Autodesk Fusion 360 part; units mm, degrees
(part 2 of 2)
sketch "스케치7" plane through (0, 0, -15.8) normal (0, 0, 1) x (-1, 0, 0) in component "right-body"
  arc A0 (-30.595085, -3.272852) -> (-28.095085, -5.772852) centre (-28.095085, -3.272852) ccw
  line L0 (-30.595085, -3.272852) -> (-218.195, -3.272852)
  arc A1 (-220.695, -5.772852) -> (-218.195, -3.272852) centre (-220.695, -3.272852) ccw
  line L1 (-220.695, -5.772852) -> (-220.695, -98.121)
  arc A2 (-218.195, -100.621) -> (-220.695, -98.121) centre (-220.695, -100.621) ccw
  line L2 (-218.195, -100.621) -> (-30.595085, -100.621)
  arc A3 (-28.095085, -98.121) -> (-30.595085, -100.621) centre (-28.095085, -100.621) ccw
  line L3 (-28.095085, -98.121) -> (-28.095085, -5.772852)
  line L4 (-30.595085, -100.621) -> (-30.595085, -3.272852)
  line L5 (-33.595085, -87.321) -> (-45.595085, -87.321)
  line L6 (-45.595085, -87.321) -> (-45.595085, -84.321)
  line L7 (-45.595085, -84.321) -> (-33.595085, -84.321)
  line L8 (-33.595085, -84.321) -> (-33.595085, -87.321)
  line L9 (-218.195, -100.621) -> (-30.595085, -100.621)
  line L10 (-58.595085, -65.221) -> (-76.595085, -65.221)
  line L11 (-76.595085, -65.221) -> (-76.595085, -62.221)
  line L12 (-76.595085, -62.221) -> (-58.595085, -62.221)
  line L13 (-58.595085, -62.221) -> (-58.595085, -65.221)
  line L14 (-59.9071, -58.8987) -> (-59.9071, -44.9972)
  line L15 (-65.0569, -44.9972) -> (-65.0569, -58.8987)
  line L16 (-78.957, -58.8987) -> (-78.957, -44.9972)
  line L17 (-84.1069, -44.9972) -> (-84.1069, -58.8987)
  line L18 (-98.007, -58.8987) -> (-98.007, -44.9972)
  line L19 (-103.1569, -44.9972) -> (-103.1569, -58.8987)
  line L20 (-117.057, -58.8987) -> (-117.057, -44.9972)
  line L21 (-122.2069, -44.9972) -> (-122.2069, -58.8987)
  line L22 (-136.107, -58.8987) -> (-136.107, -44.9972)
  line L23 (-141.257, -44.9972) -> (-141.257, -58.8987)
  line L24 (-155.157, -58.8987) -> (-155.157, -44.9972)
  line L25 (-165.662, -44.2475) -> (-165.662, -58.3477)
  line L26 (-59.9071, -51.94795) -> (-65.0569, -51.94795)
  line L27 (-78.957, -51.94795) -> (-84.1069, -51.94795)
  line L28 (-98.007, -51.94795) -> (-103.1569, -51.94795)
  line L29 (-117.057, -51.94795) -> (-122.2069, -51.94795)
  line L30 (-136.107, -51.94795) -> (-141.257, -51.94795)
  line L31 (-155.157, -51.94795) -> (-165.662, -51.94795)
  line L32 (-63.982, -53.44795) -> (-60.982, -53.44795)
  line L33 (-60.982, -53.44795) -> (-60.982, -50.44795)
  line L34 (-60.982, -50.44795) -> (-63.982, -50.44795)
  line L35 (-63.982, -50.44795) -> (-63.982, -53.44795)
  line L36 (-63.982, -53.44795) -> (-60.982, -50.44795) construction
  line L37 (-60.982, -53.44795) -> (-63.982, -50.44795) construction
  line L38 (-83.03195, -53.44795) -> (-80.03195, -53.44795)
  line L39 (-80.03195, -53.44795) -> (-80.03195, -50.44795)
  line L40 (-80.03195, -50.44795) -> (-83.03195, -50.44795)
  line L41 (-83.03195, -50.44795) -> (-83.03195, -53.44795)
  line L42 (-83.03195, -53.44795) -> (-80.03195, -50.44795) construction
  line L43 (-80.03195, -53.44795) -> (-83.03195, -50.44795) construction
  line L44 (-102.08195, -53.44795) -> (-99.08195, -53.44795)
  line L45 (-99.08195, -53.44795) -> (-99.08195, -50.44795)
  line L46 (-99.08195, -50.44795) -> (-102.08195, -50.44795)
  line L47 (-102.08195, -50.44795) -> (-102.08195, -53.44795)
  line L48 (-102.08195, -53.44795) -> (-99.08195, -50.44795) construction
  line L49 (-99.08195, -53.44795) -> (-102.08195, -50.44795) construction
  line L50 (-121.13195, -53.44795) -> (-118.13195, -53.44795)
  line L51 (-118.13195, -53.44795) -> (-118.13195, -50.44795)
  line L52 (-118.13195, -50.44795) -> (-121.13195, -50.44795)
  line L53 (-121.13195, -50.44795) -> (-121.13195, -53.44795)
  line L54 (-121.13195, -53.44795) -> (-118.13195, -50.44795) construction
  line L55 (-118.13195, -53.44795) -> (-121.13195, -50.44795) construction
  line L56 (-140.182, -53.44795) -> (-137.182, -53.44795)
  line L57 (-137.182, -53.44795) -> (-137.182, -50.44795)
  line L58 (-137.182, -50.44795) -> (-140.182, -50.44795)
  line L59 (-140.182, -50.44795) -> (-140.182, -53.44795)
  line L60 (-140.182, -53.44795) -> (-137.182, -50.44795) construction
  line L61 (-137.182, -53.44795) -> (-140.182, -50.44795) construction
  line L62 (-162.9095, -54.44795) -> (-157.9095, -54.44795)
  line L63 (-157.9095, -54.44795) -> (-157.9095, -49.44795)
  line L64 (-157.9095, -49.44795) -> (-162.9095, -49.44795)
  line L65 (-162.9095, -49.44795) -> (-162.9095, -54.44795)
  line L66 (-162.9095, -54.44795) -> (-157.9095, -49.44795) construction
  line L67 (-157.9095, -54.44795) -> (-162.9095, -49.44795) construction
  point P0 (-30.595085, -100.621)
  point P1 (-30.595085, -3.272852)
  point P2 (-62.482, -51.94795)
  point P3 (-81.53195, -51.94795)
  point P4 (-100.58195, -51.94795)
  point P5 (-119.63195, -51.94795)
  point P6 (-138.682, -51.94795)
  point P7 (-160.4095, -51.94795)
  dimension "d141" = 12
  dimension "d142" = 3
  dimension "d143" = 3
  dimension "d144" = 13.3
  dimension "d145" = 18
  dimension "d146" = 3
  dimension "d147" = 28
  dimension "d148" = 35.4
  dimension "d149" = 3
  dimension "d150" = 3
  dimension "d151" = 3
  dimension "d152" = 3
  dimension "d153" = 3
  dimension "d154" = 3
  dimension "d155" = 3
  dimension "d156" = 3
  dimension "d157" = 3
  dimension "d158" = 3
  dimension "d159" = 5
  dimension "d160" = 5
  constraint horizontal L5
  constraint vertical L6
  constraint horizontal L7
  constraint vertical L8
  constraint horizontal L10
  constraint vertical L11
  constraint horizontal L12
  constraint vertical L13
  constraint perpendicular L25 L31
  constraint horizontal L32
  constraint perpendicular L32 L33
  constraint parallel L32 L34
  constraint parallel L33 L35
  constraint horizontal L38
  constraint perpendicular L38 L39
  constraint parallel L38 L40
  constraint parallel L39 L41
  constraint horizontal L44
  constraint perpendicular L44 L45
  constraint parallel L44 L46
  constraint parallel L45 L47
  constraint horizontal L50
  constraint perpendicular L50 L51
  constraint parallel L50 L52
  constraint parallel L51 L53
  constraint horizontal L56
  constraint perpendicular L56 L57
  constraint parallel L56 L58
  constraint parallel L57 L59
  constraint horizontal L62
  constraint perpendicular L62 L63
  constraint parallel L62 L64
  constraint parallel L63 L65
extrude "돌출6'" add sketch "스케치7" along normal blind 15.8 contours L26 L32 L33 L35 | L26 L33 L34 L35 | L27 L38 L39 L41 | L27 L39 L40 L41 | L28 L44 L45 L47 | L28 L45 L46 L47 | L29 L50 L51 L53 | L29 L51 L52 L53 | L30 L56 L57 L59 | L30 L57 L58 L59 | L31 L62 L63 L65 | L31 L63 L64 L65 picked at (-61.982, -52.44795) picked at (-62.982, -51.44795) picked at (-82.03195, -52.94795) picked at (-81.03195, -51.44795) picked at (-101.08195, -52.94795) picked at (-100.08195, -51.44795) picked at (-120.13195, -52.44795) picked at (-119.13195, -50.94795) picked at (-139.182, -52.44795) picked at (-138.182, -51.44795) picked at (-161.242833, -52.781283) picked at (-159.576167, -51.114617) bodies 5 in component "right-body"
extrude "돌출7'" add sketch "스케치7" along normal blind 2 contours L5 L6 L7 L8 | L10 L11 L12 L13 picked at (-37.595085, -86.321) picked at (-64.595085, -64.221) bodies 5 in component "right-body"
sketch "스케치8" plane through (0, 100.621, 0) normal (0, -1, 0) x (1, 0, 0) in component "right-body"
  line L0 (30.595085, 0) -> (30.595085, -15.8)
  line L1 (218.195, -15.8) -> (30.595085, -15.8)
  circle A0 centre (37.595085, -12.4) radius 3.2
  line L2 (65.595085, -14.35) -> (71.395085, -14.35)
  arc A1 (71.395085, -14.35) -> (71.395085, -10.65) centre (71.395085, -12.5) ccw
  line L3 (71.395085, -10.65) -> (65.595085, -10.65)
  arc A2 (65.595085, -10.65) -> (65.595085, -14.35) centre (65.595085, -12.5) ccw
  line L4 (65.595085, -12.5) -> (71.395085, -12.5) construction
  line L5 (30.595085, -15.8) -> (218.195, -15.8)
  dimension "d165" = 6.4
  dimension "d166" = 7
  dimension "d167" = 3.4
  dimension "d169" = 3.7
  dimension "d170" = 3.3
  dimension "d171" = 35
  dimension "d172" = 5.8
  constraint tangent L2 A1
  constraint tangent A1 L3
  constraint parallel L2 L3
  constraint tangent L3 A2
  constraint tangent L2 A2
  constraint horizontal L4
  measures "d165" diameter of A0
  measures "d169" diameter of A1
sketch "스케치5 (2)" plane through (223.695, 0, 0) normal (1, 0, 0) x (0, 1, 0)
sketch "스케치1 (7)" plane through (223.695, 0, 0) normal (1, 0, 0) x (0, 1, 0) in component "right-palm-rest"
  line L0 (4.053877, -16.7) -> (4.053877, -17.8)
  line L1 (4.053877, -17.8) -> (99.839975, -17.8)
  line L2 (99.839975, -17.8) -> (99.839975, -16.7)
  line L3 (99.839975, -16.7) -> (100.621, -16.7)
  line L4 (100.621, -16.7) -> (100.621, 0)
  line L5 (100.621, 0) -> (3.272852, 0)
  line L6 (3.272852, 0) -> (3.272852, -16.7)
  line L7 (3.272852, -16.7) -> (4.053877, -16.7)
  line L8 (-20.880927, -17.8) -> (-100.880927, -17.8)
  line L9 (-20.880927, -17.8) -> (-20.880927, 7.2)
  line L10 (-100.880927, -17.8) -> (-100.880927, -6.972882)
  line L11 (-20.880927, 7.2) -> (-44.979228, 7.2)
  line L12 (-46.768082, 7.038699) -> (-96.775354, -2.053532)
  arc A0 (-96.775354, -2.053532) -> (-100.880927, -6.972882) centre (-95.880927, -6.972882) ccw
  arc A1 (-44.979228, 7.2) -> (-46.768082, 7.038699) centre (-44.979228, -2.8) ccw
  point P0 (-100.880927, -2.8)
  point P1 (-45.880927, 7.2)
  dimension "d195" = 80
  dimension "d196" = 25
  dimension "d197" = 15
  dimension "d198" = 25
  dimension "d199" = 5
  dimension "d200" = 10
  constraint horizontal L8
  constraint perpendicular L8 L9
  constraint perpendicular L8 L10
  constraint perpendicular L9 L11
  constraint tangent L12 A0
  constraint tangent L10 A0
  constraint tangent L11 A1
  constraint tangent L12 A1
  measures "d199" radius of A0
  measures "d200" radius of A1
extrude "돌출1'''''" add sketch "스케치1 (7)" against normal blind 198.6 separate body contours L8 L9 L10 L11 L12 A0 A1 picked at (-56.176646, -9.520434) makes body 6 in component "right-palm-rest"
draft "기울기1'" angle -10 neutral plane through (223.695, -20.880927, -17.8) pull (0, 1, 0) 1 faces at (223.695, -56.176646, -9.520434) on bodies 6 in component "right-palm-rest"
draft "기울기2'" angle -10 neutral plane through (223.695, -20.880927, -17.8) pull (0, 1, 0) 1 faces at (25.095, -56.176646, -9.520434) on bodies 6 in component "right-palm-rest"
fillet "필렛1''" radius 5 5 edges at (39.201158, -100.880927, -12.386441) (38.9964, -99.719686, -3.769145) (34.06842, -71.771718, 2.492583) (29.502532, -45.877284, 7.159593) (27.21959, -32.930078, 7.2) on bodies 6 in component "right-palm-rest"
fillet "필렛2'" radius 5 5 edges at (221.57041, -32.930078, 7.2) (219.287468, -45.877284, 7.159593) (214.72158, -71.771718, 2.492583) (209.7936, -99.719686, -3.769145) (209.588842, -100.880927, -12.386441) on bodies 6 in component "right-palm-rest"
sketch "스케치1 (8)" plane through (-33.692, 0, 0) normal (1, 0, 0) x (0, 1, 0) in component "left-palm-rest (2)"
  line L0 (-46.768082, 7.038699) -> (-96.775354, -2.053532)
  line L1 (-20.880927, 7.2) -> (-44.979228, 7.2)
  line L2 (-100.880927, -17.8) -> (-100.880927, -6.972882)
  line L3 (-20.880927, -17.8) -> (-100.880927, -17.8)
  line L4 (-20.880927, -17.8) -> (-20.880927, 7.2)
  arc A0 (-44.979228, 7.2) -> (-46.768082, 7.038699) centre (-44.979228, -2.8) ccw
  arc A1 (-96.775354, -2.053532) -> (-100.880927, -6.972882) centre (-95.880927, -6.972882) ccw
  point P0 (-95.880927, -6.972882)
  point P1 (-44.979228, -2.8)
extrude "돌출1''''''" add sketch "스케치1 (8)" against normal blind 146 separate body contours L0 L1 L2 L3 L4 A0 A1 picked at (-56.176646, -9.520434) makes body 7 in component "left-palm-rest (2)"
draft "기울기1''" angle -10 neutral plane through (-33.692, -20.880927, -17.8) pull (0, 1, 0) 1 faces at (-33.692, -56.176646, -9.520434) on bodies 7 in component "left-palm-rest (2)"
draft "기울기2''" angle -10 neutral plane through (-33.692, -20.880927, -17.8) pull (0, 1, 0) 1 faces at (-179.692, -56.176646, -9.520434) on bodies 7 in component "left-palm-rest (2)"
fillet "필렛1'''" radius 5 5 edges at (-165.585842, -100.880927, -12.386441) (-165.7906, -99.719686, -3.769145) (-170.71858, -71.771718, 2.492583) (-175.284468, -45.877284, 7.159593) (-177.56741, -32.930078, 7.2) on bodies 7 in component "left-palm-rest (2)"
fillet "필렛1'''" radius 5 5 edges at (-35.81659, -32.930078, 7.2) (-38.099532, -45.877284, 7.159593) (-42.66542, -71.771718, 2.492583) (-47.5934, -99.719686, -3.769145) (-47.798158, -100.880927, -12.386441) on bodies 7 in component "left-palm-rest (2)"
sketch "스케치3 (4)" plane through (0, 0, 0) normal (0, 0, -1) x (1, 0, 0) in component "left-switch"
  line L0 (-72.674, -20.2475) -> (-69.474, -20.2475)
  line L1 (-72.674, -6.14744) -> (-72.674, -20.2475)
  line L2 (-69.474, -20.2475) -> (-69.474, -6.14744)
  line L3 (-69.474, -6.14744) -> (-72.674, -6.14744)
  line L4 (-45.674, -6.14744) -> (-48.874, -6.14744)
  line L5 (-45.674, -20.2475) -> (-45.674, -6.14744)
  line L6 (-48.874, -6.14744) -> (-48.874, -20.2475)
  line L7 (-48.874, -20.2475) -> (-45.674, -20.2475)
  line L8 (-164.7244, -25.1974) -> (-167.9242, -25.1974)
  line L9 (-167.9242, -25.1974) -> (-167.9242, -39.2977)
  line L10 (-164.7244, -39.2977) -> (-164.7244, -25.1974)
  line L11 (-167.9242, -39.2977) -> (-164.7244, -39.2977)
  line L12 (-144.1243, -39.2977) -> (-140.9242, -39.2977)
  line L13 (-144.1243, -25.1974) -> (-144.1243, -39.2977)
  line L14 (-140.9242, -39.2977) -> (-140.9242, -25.1974)
  line L15 (-140.9242, -25.1974) -> (-144.1243, -25.1974)
  line L16 (-167.9242, -25.1974) -> (-164.7244, -25.1974)
  line L17 (-164.7244, -25.1974) -> (-164.7244, -23.9974)
  line L18 (-164.7244, -23.9974) -> (-167.9242, -23.9974)
  line L19 (-167.9242, -23.9974) -> (-167.9242, -25.1974)
  line L20 (-167.9242, -39.2977) -> (-164.7244, -39.2977)
  line L21 (-164.7244, -39.2977) -> (-164.7244, -40.4977)
  line L22 (-164.7244, -40.4977) -> (-167.9242, -40.4977)
  line L23 (-167.9242, -40.4977) -> (-167.9242, -39.2977)
  line L24 (-144.1243, -25.1974) -> (-140.9242, -25.1974)
  line L25 (-140.9242, -25.1974) -> (-140.9242, -23.9974)
  line L26 (-140.9242, -23.9974) -> (-144.1243, -23.9974)
  line L27 (-144.1243, -23.9974) -> (-144.1243, -25.1974)
  line L28 (-144.1243, -39.2977) -> (-140.9242, -39.2977)
  line L29 (-140.9242, -39.2977) -> (-140.9242, -40.4977)
  line L30 (-140.9242, -40.4977) -> (-144.1243, -40.4977)
  line L31 (-144.1243, -40.4977) -> (-144.1243, -39.2977)
  line L32 (-72.674, -6.14744) -> (-69.474, -6.14744)
  line L33 (-69.474, -6.14744) -> (-69.474, -4.94744)
  line L34 (-69.474, -4.94744) -> (-72.674, -4.94744)
  line L35 (-72.674, -4.94744) -> (-72.674, -6.14744)
  line L36 (-72.674, -20.2475) -> (-69.474, -20.2475)
  line L37 (-69.474, -20.2475) -> (-69.474, -21.4475)
  line L38 (-69.474, -21.4475) -> (-72.674, -21.4475)
  line L39 (-72.674, -21.4475) -> (-72.674, -20.2475)
  line L40 (-48.874, -6.14744) -> (-45.674, -6.14744)
  line L41 (-45.674, -6.14744) -> (-45.674, -4.94744)
  line L42 (-45.674, -4.94744) -> (-48.874, -4.94744)
  line L43 (-48.874, -4.94744) -> (-48.874, -6.14744)
  line L44 (-48.874, -20.2475) -> (-45.674, -20.2475)
  line L45 (-45.674, -20.2475) -> (-45.674, -21.4475)
  line L46 (-45.674, -21.4475) -> (-48.874, -21.4475)
  line L47 (-48.874, -21.4475) -> (-48.874, -20.2475)
  dimension "d223" = 1.2
  dimension "d224" = 1.2
  dimension "d225" = 1.2
  dimension "d226" = 1.2
  dimension "d227" = 1.2
  dimension "d228" = 1.2
  dimension "d229" = 1.2
  dimension "d230" = 1.2
  constraint horizontal L16
  constraint vertical L17
  constraint horizontal L18
  constraint vertical L19
  constraint coincident L8.end L9.start
  constraint horizontal L20
  constraint vertical L21
  constraint horizontal L22
  constraint vertical L23
  constraint coincident L9.end L11.start
  constraint horizontal L24
  constraint vertical L25
  constraint horizontal L26
  constraint vertical L27
  constraint coincident L13.start L15.end
  constraint horizontal L28
  constraint vertical L29
  constraint horizontal L30
  constraint vertical L31
  constraint coincident L12.start L13.end
  constraint horizontal L32
  constraint vertical L33
  constraint horizontal L34
  constraint vertical L35
  constraint horizontal L36
  constraint vertical L37
  constraint horizontal L38
  constraint vertical L39
  constraint coincident L0.start L1.end
  constraint horizontal L40
  constraint vertical L41
  constraint horizontal L42
  constraint vertical L43
  constraint horizontal L44
  constraint vertical L45
  constraint horizontal L46
  constraint vertical L47
  constraint coincident L6.end L7.start
  measures "d223" distance of L8.end L18.end
  measures "d224" distance of L9.end L22.end
  measures "d225" distance of L13.start L26.end
  measures "d226" distance of L12.start L30.end
  measures "d228" distance of L0.start L38.end
  measures "d230" distance of L6.end L46.end
extrude "돌출3''" cut sketch "스케치3 (4)" against normal blind 3.1 contours L0 L36 L37 L38 L39 | L3 L32 L33 L34 L35 | L4 L40 L41 L42 L43 | L7 L44 L45 L46 L47 | L8 L16 L17 L18 L19 | L11 L20 L21 L22 L23 | L12 L28 L29 L30 L31 | L15 L24 L25 L26 L27 picked at (-70.540667, -20.6475) picked at (-71.607333, -5.34744) picked at (-47.807333, -5.34744) picked at (-46.740667, -21.0475) picked at (-165.791, -24.7974) picked at (-166.8576, -40.0977) picked at (-143.0576, -39.6977) picked at (-143.0576, -24.3974) bodies 1 in component "left-switch"
sketch "스케치3 (5)" plane through (0, 0, 0) normal (0, 0, -1) x (1, 0, 0) in component "right-switch"
  line L0 (170.045, -82.3475) -> (166.844, -82.3475)
  line L1 (166.844, -96.4477) -> (170.045, -96.4477)
  line L2 (146.243, -82.3475) -> (143.044, -82.3475)
  line L3 (143.044, -96.4477) -> (146.243, -96.4477)
  line L4 (164.462, -58.3477) -> (167.663, -58.3477)
  line L5 (167.663, -44.2475) -> (164.462, -44.2475)
  line L6 (143.863, -44.2475) -> (140.662, -44.2475)
  line L7 (140.662, -58.3477) -> (143.863, -58.3477)
  line L8 (67.6508, -6.14744) -> (64.4507, -6.14744)
  line L9 (43.8506, -6.14744) -> (40.6506, -6.14744)
  line L10 (40.6506, -20.2475) -> (43.8506, -20.2475)
  line L11 (170.045, -96.4477) -> (166.844, -96.4477)
  line L12 (166.844, -96.4477) -> (166.844, -97.6477)
  line L13 (166.844, -97.6477) -> (170.045, -97.6477)
  line L14 (170.045, -97.6477) -> (170.045, -96.4477)
  line L15 (170.045, -82.3475) -> (166.844, -82.3475)
  line L16 (166.844, -82.3475) -> (166.844, -81.1475)
  line L17 (166.844, -81.1475) -> (170.045, -81.1475)
  line L18 (170.045, -81.1475) -> (170.045, -82.3475)
  line L19 (146.243, -96.4477) -> (143.044, -96.4477)
  line L20 (143.044, -96.4477) -> (143.044, -97.6477)
  line L21 (143.044, -97.6477) -> (146.243, -97.6477)
  line L22 (146.243, -97.6477) -> (146.243, -96.4477)
  line L23 (146.243, -82.3475) -> (143.044, -82.3475)
  line L24 (143.044, -82.3475) -> (143.044, -81.1475)
  line L25 (143.044, -81.1475) -> (146.243, -81.1475)
  line L26 (146.243, -81.1475) -> (146.243, -82.3475)
  line L27 (167.663, -58.3477) -> (164.462, -58.3477)
  line L28 (164.462, -58.3477) -> (164.462, -59.5477)
  line L29 (164.462, -59.5477) -> (167.663, -59.5477)
  line L30 (167.663, -59.5477) -> (167.663, -58.3477)
  line L31 (167.663, -44.2475) -> (164.462, -44.2475)
  line L32 (164.462, -44.2475) -> (164.462, -43.0475)
  line L33 (164.462, -43.0475) -> (167.663, -43.0475)
  line L34 (167.663, -43.0475) -> (167.663, -44.2475)
  line L35 (143.863, -58.3477) -> (140.662, -58.3477)
  line L36 (140.662, -58.3477) -> (140.662, -59.5477)
  line L37 (140.662, -59.5477) -> (143.863, -59.5477)
  line L38 (143.863, -59.5477) -> (143.863, -58.3477)
  line L39 (143.863, -44.2475) -> (140.662, -44.2475)
  line L40 (140.662, -44.2475) -> (140.662, -43.0475)
  line L41 (140.662, -43.0475) -> (143.863, -43.0475)
  line L42 (143.863, -43.0475) -> (143.863, -44.2475)
  line L43 (67.6508, -6.14744) -> (64.4507, -6.14744)
  line L44 (64.4507, -6.14744) -> (64.4507, -4.94744)
  line L45 (64.4507, -4.94744) -> (67.6508, -4.94744)
  line L46 (67.6508, -4.94744) -> (67.6508, -6.14744)
  line L47 (43.8506, -20.2475) -> (40.6506, -20.2475)
  line L48 (40.6506, -20.2475) -> (40.6506, -21.4475)
  line L49 (40.6506, -21.4475) -> (43.8506, -21.4475)
  line L50 (43.8506, -21.4475) -> (43.8506, -20.2475)
  line L51 (43.8506, -6.14744) -> (40.6506, -6.14744)
  line L52 (40.6506, -6.14744) -> (40.6506, -4.94744)
  line L53 (40.6506, -4.94744) -> (43.8506, -4.94744)
  line L54 (43.8506, -4.94744) -> (43.8506, -6.14744)
  line L55 (64.4507, -20.2475) -> (67.6508, -20.2475)
  line L56 (67.6508, -20.2475) -> (64.4507, -20.2475)
  line L57 (64.4507, -20.2475) -> (64.4507, -21.4475)
  line L58 (64.4507, -21.4475) -> (67.6508, -21.4475)
  line L59 (67.6508, -21.4475) -> (67.6508, -20.2475)
  dimension "d233" = 1.2
  dimension "d234" = 1.2
  dimension "d235" = 1.2
  dimension "d236" = 1.2
  dimension "d237" = 1.2
  dimension "d238" = 1.2
  dimension "d239" = 1.2
  dimension "d240" = 1.2
  dimension "d242" = 1.2
  dimension "d243" = 1.2
  dimension "d244" = 1.2
  dimension "d245" = 1.2
  constraint horizontal L11
  constraint vertical L12
  constraint horizontal L13
  constraint vertical L14
  constraint coincident L1.end L11.start
  constraint horizontal L15
  constraint vertical L16
  constraint horizontal L17
  constraint vertical L18
  constraint coincident L0.start L15.start
  constraint horizontal L19
  constraint vertical L20
  constraint horizontal L21
  constraint vertical L22
  constraint coincident L3.end L19.start
  constraint horizontal L23
  constraint vertical L24
  constraint horizontal L25
  constraint vertical L26
  constraint coincident L2.start L23.start
  constraint horizontal L27
  constraint vertical L28
  constraint horizontal L29
  constraint vertical L30
  constraint coincident L4.end L27.start
  constraint horizontal L31
  constraint vertical L32
  constraint horizontal L33
  constraint vertical L34
  constraint coincident L5.start L31.start
  constraint horizontal L35
  constraint vertical L36
  constraint horizontal L37
  constraint vertical L38
  constraint coincident L7.end L35.start
  constraint horizontal L39
  constraint vertical L40
  constraint horizontal L41
  constraint vertical L42
  constraint coincident L6.start L39.start
  constraint horizontal L43
  constraint vertical L44
  constraint horizontal L45
  constraint vertical L46
  constraint horizontal L47
  constraint vertical L48
  constraint horizontal L49
  constraint vertical L50
  constraint coincident L10.end L47.start
  constraint horizontal L51
  constraint vertical L52
  constraint horizontal L53
  constraint vertical L54
  constraint horizontal L56
  constraint vertical L57
  constraint horizontal L58
  constraint vertical L59
  constraint coincident L55.end L56.start
  measures "d233" distance of L1.end L13.end
  measures "d234" distance of L0.start L17.end
  measures "d235" distance of L3.end L21.end
  measures "d236" distance of L2.start L25.end
  measures "d237" distance of L4.end L29.end
  measures "d238" distance of L5.start L33.end
  measures "d239" distance of L7.end L37.end
  measures "d240" distance of L6.start L41.end
  measures "d243" distance of L10.end L49.end
  measures "d245" distance of L55.end L58.end
extrude "돌출3'''" cut sketch "스케치3 (5)" against normal blind 3.1 contours L0 L15 L16 L17 L18 | L1 L11 L12 L13 L14 | L2 L23 L24 L25 L26 | L3 L19 L20 L21 L22 | L4 L27 L28 L29 L30 | L5 L31 L32 L33 L34 | L6 L39 L40 L41 L42 | L7 L35 L36 L37 L38 | L8 L43 L44 L45 L46 | L9 L51 L52 L53 L54 | L10 L47 L48 L49 L50 | L55 L56 L57 L58 L59 picked at (168.978, -81.9475) picked at (167.911, -96.8477) picked at (145.176667, -81.9475) picked at (144.110333, -96.8477) picked at (165.529, -58.7477) picked at (166.596, -43.8475) picked at (141.729, -43.8475) picked at (141.729, -58.7477) picked at (65.5174, -5.34744) picked at (42.783933, -5.74744) picked at (41.717267, -21.0475) picked at (65.5174, -21.0475) bodies 4 in component "right-switch"
extrude "돌출10" cut sketch "스케치8" against normal blind 8 contours A0 | L2 A1 L3 A2 picked at (39.183171, -12.9098) picked at (69.461751, -13.116667) bodies 5 in component "right-body"
sketch "스케치9" plane through (0, 103.621, 0) normal (0, 1, 0) x (-1, 0, 0) in component "right-body"
  line L0 (-65.595085, -14.35) -> (-71.395085, -14.35)
  arc A0 (-65.595085, -14.35) -> (-65.595085, -10.65) centre (-65.595085, -12.5) ccw
  line L1 (-71.395085, -10.65) -> (-65.595085, -10.65)
  arc A1 (-71.395085, -10.65) -> (-71.395085, -14.35) centre (-71.395085, -12.5) ccw
  line L2 (-71.395085, -16.25) -> (-65.595085, -16.25)
  arc A2 (-65.595085, -16.25) -> (-65.595085, -8.75) centre (-65.595085, -12.5) ccw
  line L3 (-65.595085, -8.75) -> (-71.395085, -8.75)
  arc A3 (-71.395085, -8.75) -> (-71.395085, -16.25) centre (-71.395085, -12.5) ccw
  line L4 (-71.395085, -12.5) -> (-65.595085, -12.5) construction
  dimension "d250" = 7.5
  constraint tangent L2 A2
  constraint tangent A2 L3
  constraint parallel L2 L3
  constraint tangent L3 A3
  constraint tangent L2 A3
  constraint horizontal L4
  measures "d250" diameter of A2
extrude "돌출11" cut sketch "스케치9" against normal blind 1.5 contours L2 A2 L3 A3 picked at (-69.461751, -15.616667) bodies 5 in component "right-body"
extrude "돌출8" [suppressed] in component "right-body"
sketch "스케치4 (2)" plane through (0, 103.621, 0) normal (0, 1, 0) x (-1, 0, 0)
  line L0 (-70.395085, -10.7) -> (-65.595085, -10.7)
  line L1 (-65.595085, -14.3) -> (-70.395085, -14.3)
  arc A0 (-70.395085, -10.7) -> (-70.395085, -14.3) centre (-70.395085, -12.5) ccw
  arc A1 (-65.595085, -14.3) -> (-65.595085, -10.7) centre (-65.595085, -12.5) ccw
  line L2 (-70.395085, -16.25) -> (-65.595085, -16.25)
  arc A2 (-65.595085, -16.25) -> (-65.595085, -8.75) centre (-65.595085, -12.5) ccw
  line L3 (-65.595085, -8.75) -> (-70.395085, -8.75)
  arc A3 (-70.395085, -8.75) -> (-70.395085, -16.25) centre (-70.395085, -12.5) ccw
  line L4 (-70.395085, -12.5) -> (-65.595085, -12.5) construction
  dimension "d175" = 7.5
  constraint tangent L2 A2
  constraint tangent A2 L3
  constraint parallel L2 L3
  constraint tangent L3 A3
  constraint tangent L2 A3
  constraint parallel L0 L4
  measures "d175" diameter of A2
extrude "돌출9'" [suppressed] in component "right-body"
ref_plane "작업 평면1" through (-106.7985, 51.946926, -8.9) normal (1, 0, 0) x (0, -1, 0) in component "left-palm-rest (1)"
sketch "스케치1 (9)" plane through (-106.7985, 0, 0) normal (1, 0, 0) x (0, 1, 0) in component "left-palm-rest (1)"
  line L0 (-98.705795, -19.928006) -> (-18.705795, -19.928006)
  line L1 (-18.705795, -19.928006) -> (-18.705795, -22.80737)
  line L2 (-18.705795, -22.80737) -> (-98.705795, -22.80737)
  line L3 (-98.705795, -22.80737) -> (-98.705795, -19.928006)
  line L4 (-18.705795, -19.928006) -> (-18.705795, 5.071994)
  line L5 (-18.705795, 5.071994) -> (-52.608073, 5.071994)
  line L6 (-98.705795, -19.928006) -> (-98.705795, -8.136693)
  line L7 (-95.573517, -4.231945) -> (-54.777377, 4.833864)
  arc A0 (-52.608073, 5.071994) -> (-54.777377, 4.833864) centre (-52.608073, -4.928006) ccw
  arc A1 (-95.573517, -4.231945) -> (-98.705795, -8.136693) centre (-94.705795, -8.136693) ccw
  point P0 (-53.705795, 5.071994)
  point P1 (-98.705795, -4.928006)
  dimension "d179" = 80
  dimension "d180" = 25
  dimension "d181" = 35
  dimension "d182" = 15
  dimension "d183" = 10
  dimension "d184" = 4
  constraint horizontal L0
  constraint vertical L1
  constraint horizontal L2
  constraint vertical L3
  constraint perpendicular L0 L4
  constraint perpendicular L4 L5
  constraint perpendicular L0 L6
  constraint tangent L5 A0
  constraint tangent L7 A0
  constraint tangent L7 A1
  constraint tangent L6 A1
  measures "d183" radius of A0
  measures "d184" radius of A1
extrude "돌출1'''''''" [suppressed] in component "left-palm-rest (1)"
draft "기울기1'''" [suppressed] in component "left-palm-rest (1)"
draft "기울기2'''" [suppressed] in component "left-palm-rest (1)"
fillet "필렛1''''" [suppressed] in component "left-palm-rest (1)"
component "left-body" placed x (1, 0, 0) y (0, 1, 0) z (0, 0, 1) at (0, 0, 0)
component "left-switch" placed x (1, 0, 0) y (0, 1, 0) z (0, 0, 1) at (0, 0, 0)
component "right-switch" placed x (1, 0, 0) y (0, 1, 0) z (0, 0, 1) at (25, 0, 0)
component "right-body" placed x (1, 0, 0) y (0, 1, 0) z (0, 0, 1) at (0, 0, 0)
component "right-palm-rest" placed x (1, 0, 0) y (0, 1, 0) z (0, 0, 1) at (0, 0, 0)
component "left-palm-rest (2)" placed x (1, 0, 0) y (0, 1, 0) z (0, 0, 1) at (0, 0, 0)
equation "bolt_head_hole = 6.2 mm" comment "나사 머리"
equation "bolt_body_hole = 3.55 mm" comment "나사 몸통 폭"
equation "top_cover_height = 4.5 mm" comment "키보드 커버 높이"
equation "wall_thick = 5 mm" comment "벽면 두께"
equation "bottom_height = 2 mm" comment "바닥 높이"
equation "body_height = 15.8 mm" comment "중간 높이"
equation "body_filet = 3 mm" comment "몸체 밖 라운드"
equation "bolt_head_height = 1.1 mm" comment "볼트 머리 높이"
equation "d14 = body_filet"
equation "d15 = body_filet"
equation "d16 = body_filet"
equation "d17 = body_filet"
equation "d18 = bolt_body_hole"
equation "d19 = bolt_body_hole"
equation "d20 = bolt_body_hole"
equation "d21 = bolt_body_hole"
equation "d22 = top_cover_height"
equation "d24 = bolt_head_hole"
equation "d25 = bolt_head_hole"
equation "d26 = bolt_head_hole"
equation "d27 = bolt_head_hole"
equation "d28 = -bolt_head_height"
equation "d31 = wall_thick"
equation "d32 = wall_thick"
equation "d33 = wall_thick"
equation "d34 = wall_thick"
equation "d35 = -body_height"
equation "d37 = bottom_height"
equation "d39 = bolt_head_hole"
equation "d40 = bolt_head_hole"
equation "d41 = bolt_head_hole"
equation "d42 = bolt_head_hole"
equation "d43 = -bolt_head_height"
equation "d51 = body_filet"
equation "d53 = body_filet"
equation "d854_1 = ( 1.25 * 4 * keyWidth_1 ) + ( 2.25 * keyWidth_1 ) + bodyMargin_1 * 2"
equation "keyWidth_1 = 19.05 mm"
equation "bodyMargin_1 = 4 mm"
equation "d75 = body_filet"
equation "d76 = body_filet"
equation "d77 = body_filet"
equation "d78 = body_filet"
equation "d79 = bolt_body_hole"
equation "d80 = bolt_body_hole"
equation "d81 = bolt_body_hole"
equation "d82 = bolt_body_hole"
equation "d83 = top_cover_height"
equation "d85 = bolt_head_hole"
equation "d86 = bolt_head_hole"
equation "d87 = bolt_head_hole"
equation "d88 = bolt_head_hole"
equation "d89 = -bolt_head_height"
equation "d96 = body_height"
equation "d98 = bottom_height"
equation "d101 = bolt_head_hole"
equation "d102 = bolt_head_hole"
equation "d103 = bolt_head_hole"
equation "d104 = bolt_head_hole"
equation "d105 = -bolt_head_height"
equation "d111 = body_filet"
equation "d139 = -body_height"
equation "d161 = body_height"
equation "d178 = ( -146.213 / 2 ) * 1 mm"
equation "d185 = ( 146 / 2 ) * 1 mm"
equation "stabilizer_hole_margin = 1.2 mm" comment "스테빌 걸쇠"
equation "stabilizer_hole_height = top_cover_height - 1.4 mm" comment "스테빌 안착 높이"
equation "d223 = stabilizer_hole_margin"
equation "d224 = stabilizer_hole_margin"
equation "d225 = stabilizer_hole_margin"
equation "d226 = stabilizer_hole_margin"
equation "d227 = stabilizer_hole_margin"
equation "d228 = stabilizer_hole_margin"
equation "d229 = stabilizer_hole_margin"
equation "d230 = stabilizer_hole_margin"
equation "d231 = -stabilizer_hole_height"
equation "d233 = stabilizer_hole_margin"
equation "d234 = stabilizer_hole_margin"
equation "d235 = stabilizer_hole_margin"
equation "d236 = stabilizer_hole_margin"
equation "d237 = stabilizer_hole_margin"
equation "d238 = stabilizer_hole_margin"
equation "d239 = stabilizer_hole_margin"
equation "d240 = stabilizer_hole_margin"
equation "d242 = stabilizer_hole_margin"
equation "d243 = stabilizer_hole_margin"
equation "d244 = stabilizer_hole_margin"
equation "d245 = stabilizer_hole_margin"
equation "d246 = -stabilizer_hole_height"
equation "d250 = ( 3.75 * 2 ) * 1 mm"
